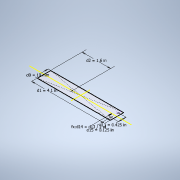
# Autodesk Inventor part: J010356
Saved by Autodesk Inventor 2020.3 (Build 243373000, 373)
## iProperties
RuleStatus: InUse
AfterDocSave0: file://Part Number Cleaner
Created: 2022-04-05
Material: POLYCARBONATE, CLEAR
Catalog Web Link: https://www.janelia.org/
Vendor: HHMI: JRC - jET
Document SubType Name: Modeling
Designer: arnoldj
Density: 1.2 g/cm^3
Appearance: Polycarbonate (Clear)
Part Number: J010356
Project: COMMON
Description: FB CHAMBER LOAD PLATE
LAB/DEPT: COMMON
REQUESTING SCIENTIST: COMMON
SURFACE ROUGHNESS: N/A
DESIGN DEPARTMENT: HHMI: JRC - jET
SPECIAL FINISH: NONE
ALTERED ITEM PART NUMBER: N/A
ALTERED ITEM VENDOR: N/A
ALTERED ITEM DESCRIPTION: N/A
Title: Standard
Author: arnoldj
Revision Number: 0
Autodesk Inventor part; units mm, degrees
ref_plane "YZ Plane" through (0, 0, 0) normal (1, 0, 0) x (0, 1, 0)
ref_plane "XZ Plane" through (0, 0, 0) normal (0, 1, 0) x (-1, 0, 0)
ref_plane "XY Plane" through (0, 0, 0) normal (0, 0, 1) x (1, 0, 0)
sketch "Sketch1" plane through (0, 0, 0) normal (0, 1, 0) x (-1, 0, 0)
  line L0 (0, -13.3) -> (0, 13.3) projected
  line L1 (-72.898, 0) -> (72.898, 0) projected
  line L2 (-52.07, -9.5) -> (52.07, -9.5)
  line L3 (52.07, -9.5) -> (52.07, 9.5)
  line L4 (52.07, 9.5) -> (-52.07, 9.5)
  line L5 (-52.07, 9.5) -> (-52.07, -9.5)
  line L6 (-52.07, -9.5) -> (52.07, 9.5) construction
  line L7 (52.07, -9.5) -> (-52.07, 9.5) construction
  point P0 (0, 0)
  point P1 (11.43, 0)
  point P2 (-48.895, 5.3975)
  point P3 (-48.895, -5.3975)
  dimension "d0" = 19
  dimension "d1" = 104.14
  dimension "d2" = 40.64
  dimension "d13" = 10.795
  dimension "d14" = 5.3975
  dimension "d15" = 3.175
  constraints: 12 end point, 2 midpoint, 2 parallel, 1 horizontal, 1 perpendicular, 1 point on line
  measures "d0" distance of L2.end L3.end
  measures "d1" distance of L3.end L4.end
  measures "d2" distance from line of point (11.43, 0) L3
  measures "d13" distance of point (-48.895, -5.397) point (-48.895, 5.397)
  measures "d14" distance from line of L1 point (-48.895, 5.397)
  measures "d15" distance from line of point (-48.895, 5.397) L5
extrude "Extrusion1" add sketch "Sketch1" against normal blind 0.762
hole "Hole1" at (-11.43, 0, 0) direction (0, -1, 0) diameter 1.7145 end through all
fillet "Fillet1" radius 1.905 4 edges at (-52.07, -0.381, 9.5) (-52.07, -0.381, -9.5) (52.07, -0.381, 9.5) (52.07, -0.381, -9.5)
hole "Hole2" at (48.895, 0, 5.3975) at (48.895, 0, -5.3975) direction (0, -1, 0) diameter 1.778 end through all countersink diameter 3.0226 countersink angle 82 clearance for "Flat Head Machine Screw (82)" size "#0" standard "Ansi Unified Screw Threads"
sketch "Sketch3" plane through (0, 0, 0) normal (0, 1, 0) x (-1, 0, 0)
  line L0 (0, -2.6111) -> (0, 15.6667) projected
  line L1 (-44.958, 0) -> (7.493, 0) projected
  circle A0 centre (-35.052, 10.6426) radius 2.413
  point P0 (0, 0)
  dimension "d26" = 4.826
  dimension "d27" = 35.052
  dimension "d28" = 10.6426
  constraints: 1 centre point
  measures "d26" diameter of A0
  measures "d27" distance from line of A0.centre L0
  measures "d28" distance from line of A0.centre L1
extrude "Extrusion2" cut sketch "Sketch3" against normal through all
mirror "Mirror2" about plane through (0, 0, 0) normal (0, 0, 1) of "Extrusion2"
fillet "Fillet2" radius 0.635 4 edges at (32.9267, -0.381, -9.5) (37.1773, -0.381, -9.5) (37.1773, -0.381, 9.5) (32.9267, -0.381, 9.5)
equation "\"d14\" = 0.5 * d13"
body "Solid1"
